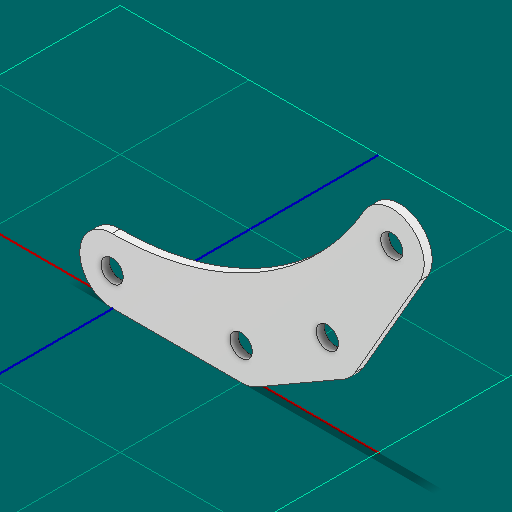
# Autodesk Inventor part: 60 Degree Gusset
Saved by Autodesk Inventor 2025 (Build 290162000, 162)
## iProperties
Created: 2024-10-22
Part Number: 60 Degree Gusset
Material: Acetal Resin, White
Document SubType Name: Modeling
Designer: averey
Density: 1.425 g/cm^3
Appearance: Smooth - White
Author: averey
Autodesk Inventor part; units mm, degrees
ref_plane "YZ Plane" through (0, 0, 0) normal (1, 0, 0) x (0, 1, 0)
ref_plane "XZ Plane" through (0, 0, 0) normal (0, 1, 0) x (-1, 0, 0)
ref_plane "XY Plane" through (0, 0, 0) normal (0, 0, 1) x (1, 0, 0)
sketch "main" plane through (0, 0, 0) normal (0, 0, 1) x (1, 0, 0)
  circle A0 centre (-6.1105, -12.0036) radius 2.1844
  circle A1 centre (-31.5105, -12.0036) radius 2.1844
  circle A2 centre (10.8754, -2.1968) radius 2.1844
  circle A3 centre (23.5754, 19.8003) radius 2.1844
  arc A4 (-31.5236, -5.6536) -> (-31.5105, -18.3536) centre (-31.5105, -12.0036) ccw
  arc A5 (-6.1105, -18.3536) -> (-2.9355, -17.5028) centre (-6.1105, -12.0036) ccw
  arc A6 (14.0504, -7.696) -> (16.3746, -5.3718) centre (10.8754, -2.1968) ccw
  arc A7 (29.0746, 16.6253) -> (18.0827, 22.9866) centre (23.5754, 19.8003) ccw
  arc A8 (-31.5236, -5.6536) -> (18.0827, 22.9866) centre (-31.6424, 51.8327) ccw
  line L0 (-31.5105, -18.3536) -> (-6.1105, -18.3536)
  line L1 (29.0746, 16.6253) -> (16.3746, -5.3718)
  line L2 (-2.9355, -17.5028) -> (14.0504, -7.696)
  point P0 (-0.7926, -1.6009)
  dimension "d0" = 12.7
  dimension "d1" = 12.7
  dimension "d2" = 12.7
  dimension "d3" = 12.7
  measures "d0" diameter of A4
  measures "d1" diameter of A5
  measures "d2" diameter of A6
  measures "d3" diameter of A7
sketch "Sketch1" plane through (0, 0, 0) normal (0, 0, 1) x (1, 0, 0)
  circle A0 centre (25.4, 0) radius 2.1844
  circle A1 centre (0, 0) radius 2.1844
  circle A2 centre (42.3858, 9.8068) radius 2.1844
  circle A3 centre (55.0858, 31.8038) radius 2.1844
  arc A4 (-0.0131, 6.35) -> (0, -6.35) centre (0, 0) ccw
  arc A5 (25.4, -6.35) -> (28.575, -5.4993) centre (25.4, 0) ccw
  arc A6 (45.5608, 4.3075) -> (47.8851, 6.6318) centre (42.3858, 9.8068) ccw
  arc A7 (60.5851, 28.6288) -> (49.5932, 34.9902) centre (55.0858, 31.8038) ccw
  arc A8 (-0.0131, 6.35) -> (49.5932, 34.9902) centre (-0.132, 63.8362) ccw
  line L0 (0, -6.35) -> (25.4, -6.35)
  line L1 (60.5851, 28.6288) -> (47.8851, 6.6318)
  line L2 (28.575, -5.4993) -> (45.5608, 4.3075)
  constraints: 1 other
extrude "Extrusion1" add sketch "Sketch1" along normal blind 1.5875
body "Solid1"
